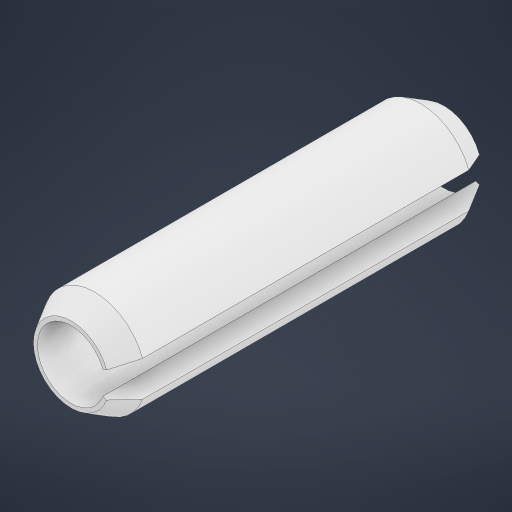
# Autodesk Inventor part: Part5
Saved by Autodesk Inventor 2023 (Build 270158000, 158)
## iProperties
Created: 2022-11-23
Part Number: Part5
Material: ABS Plastic
Document SubType Name: Modeling
Designer: iusti
Mass: 0.122658 g
Surface Area: 3.51701 cm^2
Volume: 0.115715 cm^3
Density: 1.06 g/cm^3
Appearance: Smooth - White
Author: iusti
Autodesk Inventor part; units mm, degrees
ref_plane "YZ Plane" through (0, 0, 0) normal (1, 0, 0) x (0, 1, 0)
ref_plane "XZ Plane" through (0, 0, 0) normal (0, 1, 0) x (-1, 0, 0)
ref_plane "XY Plane" through (0, 0, 0) normal (0, 0, 1) x (1, 0, 0)
sketch "Sketch1" plane through (0, 0, 0) normal (0, 0, 1) x (1, 0, 0)
  arc A0 (2.0651, 0.7586) -> (2.0651, -0.7586) centre (0, 0) ccw
  arc A1 (1.3611, 0.5) -> (1.3611, -0.5) centre (0, 0) ccw
  line L0 (2.0651, 0.7586) -> (1.3611, 0.5)
  line L1 (0, 0) -> (1.3611, -0.5) construction
  line L2 (1.3611, 0.5) -> (0, 0) construction
  line L3 (1.3611, -0.5) -> (2.0651, -0.7586)
  line L4 (-3.053, 0) -> (2.9181, 0) construction
  dimension "d0" = 4.4
  dimension "d1" = 2.9
  dimension "d2" = 1
  constraints: 8 end point, 4 point on circle, 2 centre point, 2 coincident, 2 collinear, 1 other
  measures "d0" diameter of A0
  measures "d1" diameter of A1
  measures "d2" distance of L1.end L0.end
extrude "Extrusion1" add sketch "Sketch1" along normal mid plane 16
chamfer "Chamfer1" distance 1 angle 30 2 edges at (-2.2, 0, 8) (-2.2, 0, -8) measured on face at (-1.7005, -1.3958, -2.6667)
body "Solid1"
